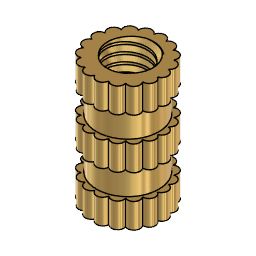
M4_10_mm_brass_thread_insert (Autodesk Fusion 360 design; units mm, degrees)
part number: 2026-06-20-09-24-02-047
Autodesk Fusion 360 part; units mm, degrees
sketch "Brass thread outline" plane through (0, 0, 0) normal (0, 0, 1) x (1, 0, 0)
  circle A0 centre (0, 0) radius 2.5
  dimension "d4" = 5
  constraint coincident A0.centre origin
  measures "d4" diameter of A0
extrude "Extrude1" add sketch "Brass thread outline" along normal blind 10
sketch "Ridges" plane through (0, 0, 10) normal (0, 0, 1) x (-1, 0, 0)
  circle A0 centre (0, 0) radius 2.5
  circle A1 centre (0, 0) radius 3
  circle A2 centre (-0.0001, -2.5) radius 0.5
  circle A3 centre (0.903, -2.3312) radius 0.5
  circle A4 centre (1.6842, -1.8476) radius 0.5
  circle A5 centre (2.2379, -1.1144) radius 0.5
  circle A6 centre (2.4893, -0.2308) radius 0.5
  circle A7 centre (2.4046, 0.6841) radius 0.5
  circle A8 centre (1.9951, 1.5065) radius 0.5
  circle A9 centre (1.3162, 2.1255) radius 0.5
  circle A10 centre (0.4595, 2.4574) radius 0.5
  circle A11 centre (-0.4593, 2.4575) radius 0.5
  circle A12 centre (-1.316, 2.1256) radius 0.5
  circle A13 centre (-1.995, 1.5067) radius 0.5
  circle A14 centre (-2.4045, 0.6843) radius 0.5
  circle A15 centre (-2.4893, -0.2306) radius 0.5
  circle A16 centre (-2.238, -1.1143) radius 0.5
  circle A17 centre (-1.6843, -1.8475) radius 0.5
  circle A18 centre (-0.9032, -2.3311) radius 0.5
  dimension "d8" = 6
  dimension "d29" = 0.0001
  dimension "d31" = 360
  constraint coincident A0.centre A1.centre
  constraint coincident A0 A2.centre
  constraint tangent A1 A2
  measures "d8" diameter of A1
  measures "d29" horizontal distance of A0.centre A2.centre
extrude "Extrude2" add sketch "Ridges" against normal blind 2 contours A0 A5 A6 A7 | A0 A5 A6 A7 | A0 A6 A7 | A0 A6 A7 | A0 A5 A6 | A0 A5 A6 | A0 A6 A7 A8 | A0 A6 A7 A8 | A2 A3 A4 A5 A6 A7 A8 A9 A10 A11 A12 A13 A14 A15 A16 A17 A18 | A0 A4 A5 A6 | A0 A4 A5 A6 | A0 A7 A8 | A0 A7 A8 | A0 A7 A8 A9 | A0 A4 A5 | A0 A4 A5 | A0 A3 A4 A5 | A0 A7 A8 A9 | A0 A8 A9 A10 | A0 A8 A9 | A0 A3 A4 A5 | A0 A2 A3 A4 | A0 A3 A4 | A0 A8 A9 | A0 A8 A9 A10 | A0 A9 A10 A11 | A0 A9 A10 | A0 A3 A4 | A0 A2 A3 A18 | A0 A2 A3 | A0 A2 A3 A4 | A0 A9 A10 | A0 A9 A10 A11 | A0 A10 A11 A12 | A0 A10 A11 | A0 A2 A3 | A0 A2 A18 | A0 A2 A17 A18 | A0 A2 A3 A18 | A0 A10 A11 | A0 A10 A11 A12 | A0 A11 A12 A13 | A0 A11 A12 | A0 A2 A17 A18 | A0 A2 A18 | A0 A16 A17 A18 | A0 A17 A18 | A0 A11 A12 | A0 A11 A12 A13 | A0 A12 A13 A14 | A0 A12 A13 | A0 A17 A18 | A0 A16 A17 A18 | A0 A12 A13 | A0 A12 A13 A14 | A0 A15 A16 A17 | A0 A16 A17 | A0 A16 A17 | A0 A13 A14 | A0 A13 A14 | A0 A13 A14 A15 | A0 A15 A16 A17 | A0 A13 A14 A15 | A0 A14 A15 A16 | A0 A15 A16 | A0 A14 A15 A16 | A0 A15 A16 | A0 A14 A15 | A0 A14 A15
pattern_linear "R-Pattern1" count 3 spacing 4 along (0, 0, -1) of "Extrude2"
sketch "Thread hole" plane through (0, 0, 10) normal (0, 0, 1) x (-1, 0, 0)
  circle A0 centre (0, 0) radius 2
  arc A1 (0.4877, -2.6097) -> (1.3975, -2.2573) centre (0.903, -2.3312) ccw
  arc A2 (1.3975, -2.2573) -> (2.1186, -1.6) centre (1.6842, -1.8476) ccw
  arc A3 (2.1186, -1.6) -> (2.5535, -0.7266) centre (2.2379, -1.1144) ccw
  arc A4 (2.5535, -0.7266) -> (2.6435, 0.2449) centre (2.4893, -0.2308) ccw
  arc A5 (2.6435, 0.2449) -> (2.3766, 1.1833) centre (2.4046, 0.6841) ccw
  arc A6 (2.3766, 1.1833) -> (1.7886, 1.9619) centre (1.9951, 1.5065) ccw
  arc A7 (1.7886, 1.9619) -> (0.9591, 2.4755) centre (1.3162, 2.1255) ccw
  arc A8 (0.9591, 2.4755) -> (0.0001, 2.6549) centre (0.4595, 2.4574) ccw
  arc A9 (0.0001, 2.6549) -> (-0.9589, 2.4756) centre (-0.4593, 2.4575) ccw
  arc A10 (-0.9589, 2.4756) -> (-1.7885, 1.962) centre (-1.316, 2.1256) ccw
  arc A11 (-1.7885, 1.962) -> (-2.3765, 1.1835) centre (-1.995, 1.5067) ccw
  arc A12 (-2.3765, 1.1835) -> (-2.6435, 0.2451) centre (-2.4045, 0.6843) ccw
  arc A13 (-2.6435, 0.2451) -> (-2.5535, -0.7264) centre (-2.4893, -0.2306) ccw
  arc A14 (-2.5535, -0.7264) -> (-2.1187, -1.5998) centre (-2.238, -1.1143) ccw
  arc A15 (-0.4879, -2.6096) -> (0.4877, -2.6097) centre (-0.0001, -2.5) ccw
  arc A16 (-2.1187, -1.5998) -> (-1.3977, -2.2571) centre (-1.6843, -1.8475) ccw
  arc A17 (-1.3977, -2.2571) -> (-0.4879, -2.6096) centre (-0.9032, -2.3311) ccw
  dimension "d11" = 4
  constraint coincident A0.centre origin
  measures "d11" diameter of A0
extrude "Extrude3" cut sketch "Thread hole" against normal blind 10 contours A0
thread "Thread2" "ISO Metric profile 4.0 M4x0.7 M4x0.7 6H" major diameter 4.1095 minor diameter 3.332 pitch 0.7 angle 60 modelled right hand crest width 0.193 on face at (-1.9975, 0.0997, 3.3333) crest through (-1.666, 0, 9.825)
equation "outer_diameter = 5 mm" comment "The outer diameter of the non-ridged parts."
equation "hole_diameter = 4 mm" comment "The thread diameter of the brass insert. 4 mm for this M4 insert."
equation "height = 10 mm" comment "The height of the brass thread insert. 10 mm for this model."
equation "d4 = outer_diameter"
equation "d5 = height"
equation "ridge_diameter = 6 mm" comment "The outer diameter of the ridged parts."
equation "d8 = ridge_diameter"
equation "d9 = -ridge_height"
equation "d11 = hole_diameter"
equation "d12 = -height"
equation "number_of_ridges = 3" comment "The number of ridges to have along the outside."
equation "d23 = number_of_ridges"
equation "d25 = -ridge_pattern_length"
equation "ridge_pattern_length = height - ridge_height" comment "The distance to use for the rectangular pattern that repeats the ridges."
equation "ridge_height = 2 mm" comment "The height of the individual ridges."
named bodies: "M4 10 mm Brass Thread Insert"
